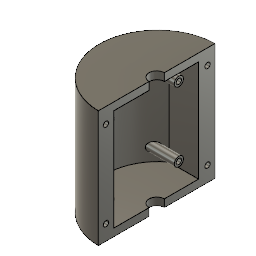
Robot Shell 3in Diameter v1 (Autodesk Fusion 360 design; units mm, degrees)
Autodesk Fusion 360 part; units mm, degrees
sketch "Sketch1" plane through (0, 0, 0) normal (0, 1, 0) x (1, 0, 0)
  circle A0 centre (0, 0) radius 38.1
  dimension "d1" = 76.2
  constraint coincident A0.centre origin
  measures "d1" diameter of A0
extrude "Extrude1" add sketch "Sketch1" along normal blind 76.2
sketch "Sketch2" plane through (0, 76.2, 0) normal (0, 1, 0) x (-1, 0, 0)
  circle A0 centre (0, 0) radius 38.1
  circle A1 centre (0, 0) radius 33.655
  line L0 (0.6095, -38.0951) -> (0.6095, 38.0951)
  dimension "d5" = 67.31
  constraint coincident A0.centre A1.centre
  constraint coincident A0 L0.start
  constraint coincident A0 L0.end
  constraint vertical L0
  measures "d5" diameter of A1
extrude "Extrude2" cut sketch "Sketch2" against normal blind 85 contours A0 A1 L0 | A1 L0 | A1 L0 picked at (-2.8347, -36.423)
sketch "Sketch3" plane through (-0.6095, 0, 0) normal (1, 0, 0) x (0, 0, -1)
  line L0 (33.6495, 0) -> (38.0951, 0)
  line L1 (38.0951, 0) -> (38.0951, 76.2)
  line L2 (38.0951, 76.2) -> (33.6495, 76.2)
  line L3 (33.6495, 76.2) -> (33.6495, 0)
  circle A0 centre (22.4126, 58.6067) radius 3
  circle A1 centre (22.4126, 13.3947) radius 3
  circle A2 centre (-22.7994, 13.3947) radius 3
  circle A3 centre (-22.7994, 58.6067) radius 3
  circle A4 centre (-22.7994, 58.6067) radius 1.75
  circle A5 centre (22.4126, 58.6067) radius 1.75
  circle A6 centre (22.4126, 13.3947) radius 1.75
  circle A7 centre (-22.7994, 13.3947) radius 1.75
  point P0 (22.4126, 58.6067)
  dimension "d11" = 6
  dimension "d12" = 6
  dimension "d13" = 6
  dimension "d14" = 6
  dimension "d15" = 3.5
  dimension "d16" = 3.5
  dimension "d17" = 3.5
  dimension "d18" = 3.5
  constraint concentric A3 A4
  constraint coincident P0 A0.centre
  constraint concentric A1 A6
  constraint concentric A2 A7
  measures "d11" diameter of A0
  measures "d12" diameter of A1
  measures "d13" diameter of A2
  measures "d14" diameter of A3
  measures "d15" diameter of A4
  measures "d16" diameter of A5
  measures "d17" diameter of A6
  measures "d18" diameter of A7
extrude "Extrude3" add sketch "Sketch3" against normal blind 27 contours A0 | A1 | A2 | A3
extrude "Extrude4" cut 4 faces at (-0.6095, 58.4576, -19.8404) (-0.6095, 13.1587, -24.9782) (-0.6095, 13.2456, 20.2273) (-0.6095, 58.3707, 20.2338) along direction (-1, 0, 0) blind 8
sketch "Sketch4" plane through (0, 76.2, 0) normal (0, 1, 0) x (-1, 0, 0)
  line L0 (0.6095, -33.6495) -> (0.6095, -38.0951)
  arc A0 (0.6095, -38.0951) -> (0.6095, 38.0951) centre (0, 0) ccw
  line L1 (0.6095, 38.0951) -> (0.6095, 33.6495)
  arc A1 (0.6095, -33.6495) -> (0.6095, 33.6495) centre (0, 0) ccw
  circle A2 centre (0, 0) radius 33.655
  line L2 (0.6095, -33.6495) -> (0.6095, 33.6495)
  constraint coincident A0.centre A1.centre
  constraint coincident L0.start A2
  constraint coincident L0.start A1.start
  constraint coincident L1.end A1.end
extrude "Extrude5" add sketch "Sketch4" against normal blind 5 contours A1 A2 L2
sketch "Sketch5" plane through (0, 0, 0) normal (0, -1, 0) x (1, 0, 0)
  line L0 (-0.6095, -38.0951) -> (-0.6095, -33.6495)
  arc A0 (-0.6095, 33.6495) -> (-0.6095, -33.6495) centre (0, 0) ccw
  line L1 (-0.6095, 33.6495) -> (-0.6095, 38.0951)
  arc A1 (-0.6095, 38.0951) -> (-0.6095, -38.0951) centre (0, 0) ccw
  circle A2 centre (0, 0) radius 33.655
  line L2 (-0.6095, 33.6495) -> (-0.6095, -33.6495)
  constraint concentric A0 A2
  constraint coincident A0.start A2
  constraint coincident A0.start L1.start
  constraint coincident L0.end A0.end
extrude "Extrude6" add sketch "Sketch5" against normal blind 5 contours A0 A2 L2
sketch "Sketch6" plane through (0, 76.2, 0) normal (0, 1, 0) x (-1, 0, 0)
  line L0 (0.6095, 38.0951) -> (0.6095, -38.0951)
  arc A0 (0.6095, -38.0951) -> (0.6095, 38.0951) centre (0, 0) ccw
  circle A1 centre (0.6095, 0) radius 5
  dimension "d28" = 10
  constraint midpoint L0 A1.centre
  measures "d28" diameter of A1
extrude "Extrude7" cut sketch "Sketch6" against normal blind 15 contours L0 A1 picked at (1.9381, 1.2426)
sketch "Sketch7" plane through (0, 0, 0) normal (0, -1, 0) x (1, 0, 0)
  line L0 (-0.6095, -38.0951) -> (-0.6095, 38.0951)
  arc A0 (-0.6095, 38.0951) -> (-0.6095, -38.0951) centre (0, 0) ccw
  circle A1 centre (-0.6095, 0) radius 5
  dimension "d31" = 10
  constraint midpoint L0 A1.centre
  measures "d31" diameter of A1
extrude "Extrude8" cut sketch "Sketch7" against normal blind 9 contours L0 A1 picked at (-2.4663, 1.3868)
sketch "Sketch8" plane through (-0.6095, 0, 0) normal (1, 0, 0) x (0, 0, -1)
  line L0 (-5, 0) -> (-5, 5)
  line L1 (-5, 5) -> (-33.6495, 5)
  line L2 (-33.6495, 5) -> (-33.6495, 71.2)
  line L3 (-33.6495, 71.2) -> (-5, 71.2)
  line L4 (-5, 71.2) -> (-5, 76.2)
  line L5 (-5, 76.2) -> (-38.0951, 76.2)
  line L6 (-38.0951, 76.2) -> (-38.0951, 0)
  line L7 (-38.0951, 0) -> (-5, 0)
  line L8 (-33.6495, 71.2) -> (-28.0413, 71.2)
  line L9 (-28.0413, 71.2) -> (-28.0413, 5)
  line L10 (-28.0413, 5) -> (-33.6495, 5)
  line L11 (-33.6495, 5) -> (-33.6495, 71.2)
  line L12 (35, 5) -> (27.216, 5)
  line L13 (27.216, 5) -> (27.216, 71.2)
  line L14 (27.216, 71.2) -> (35, 71.2)
  line L15 (35, 71.2) -> (35, 5)
  constraint horizontal L8
  constraint vertical L9
  constraint horizontal L10
  constraint vertical L11
  constraint coincident L1 L9.end
  constraint coincident L2.end L3.start
  constraint horizontal L12
  constraint vertical L13
  constraint horizontal L14
  constraint vertical L15
extrude "Extrude9" add sketch "Sketch8" against normal blind 60 contours L1 L2 L3 L8 L9 L10 L11 | L12 L13 L14 L15
sketch "Sketch9" plane through (0, 0, 0) normal (0, -1, 0) x (1, 0, 0)
  arc A0 (-0.6095, 5) -> (-0.6095, -5) centre (-0.6095, 0) ccw
  line L0 (-0.6095, 5) -> (-0.6095, 38.0951)
  arc A1 (-0.6095, 38.0951) -> (-0.6095, -38.0951) centre (0, 0) ccw
  line L1 (-0.6095, -38.0951) -> (-0.6095, -5)
  circle A2 centre (-0.6095, 0) radius 37.4984
  circle A3 centre (-0.6095, 0) radius 75.0596
  constraint concentric A0 A2
  constraint concentric A2 A3
extrude "Extrude10" cut sketch "Sketch9" against normal blind 110
sketch "Sketch10" plane through (-0.6095, 0, 0) normal (1, 0, 0) x (0, 0, -1)
  line L0 (-38.0951, 0) -> (-5, 0)
  line L1 (-5, 0) -> (-5, 5)
  line L2 (-5, 5) -> (-28.0413, 5)
  line L3 (-28.0413, 5) -> (-28.0413, 71.2)
  line L4 (-28.0413, 71.2) -> (-5, 71.2)
  line L5 (-5, 71.2) -> (-5, 76.2)
  line L6 (-5, 76.2) -> (-38.0951, 76.2)
  line L7 (-38.0951, 76.2) -> (-38.0951, 0)
  circle A0 centre (-33.0951, 10) radius 1.75
  circle A1 centre (-33.0951, 66.151) radius 1.75
  circle A2 centre (-33.0951, 66.151) radius 1.75
  circle A3 centre (-33.0951, 10) radius 1.75
  circle A4 centre (33.1, 10) radius 1.75
  circle A5 centre (33.1, 66.2) radius 1.75
  dimension "d38" = 3.5
  dimension "d43" = 3.5
  dimension "d44" = 3.5
  dimension "d45" = 3.5
  dimension "d48" = 3.5
  dimension "d51" = 3.5
  measures "d38" diameter of A0
  measures "d43" diameter of A1
  measures "d44" diameter of A3
  measures "d45" diameter of A2
  measures "d48" diameter of A4
  measures "d51" diameter of A5
extrude "Extrude11" cut sketch "Sketch10" against normal blind 6 contours A0 A3 | A1 A2 | A4 | A5
